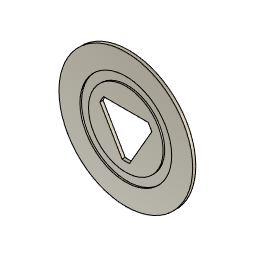
零件1 v3 (Autodesk Fusion 360 design; units mm, degrees)
Autodesk Fusion 360 part; units mm, degrees
sketch "草图1" plane through (0, 0, 0) normal (0, 1, 0) x (1, 0, 0)
  circle A0 centre (0, 0) radius 24.125
  circle A1 centre (0, 0) radius 29.375
  dimension "d1" = 48.25
  dimension "d2" = 58.75
  constraint coincident A0.centre A1.centre
  measures "d1" diameter of A0
  measures "d2" diameter of A1
extrude "拉伸1" add sketch "草图1" along normal blind 0.8 makes body 1
sketch "草图2" plane through (0, 0, 0) normal (0, -1, 0) x (1, 0, 0)
  circle A0 centre (0, 0) radius 24.125
  circle A1 centre (0, 0) radius 29.375
  circle A2 centre (0, 0) radius 43
  line L0 (2.4024, -17.839) -> (16.6502, 6.839)
  line L1 (-16.6502, 6.839) -> (-2.4024, -17.839)
  arc A3 (-14.2478, 11) -> (-16.6502, 6.839) centre (0, 0) ccw
  line L2 (14.2478, 11) -> (-14.2478, 11)
  arc A4 (16.6502, 6.839) -> (14.2478, 11) centre (0, 0) ccw
  arc A5 (-2.4024, -17.839) -> (2.4024, -17.839) centre (0, 0) ccw
  dimension "d5" = 86
  constraint coincident A0.centre A1.centre
  measures "d5" diameter of A2
extrude "拉伸2" add sketch "草图2" along normal blind 2 separate body contours A2 makes body 2
extrude "拉伸3" add sketch "草图2" along normal blind 1 contours A0 | A1 bodies 1 2
extrude "拉伸4" add 1 faces at (-15.1728, -1, -7.9151) along direction (0, -1, 0) up to surface (1 mm away) on bodies 1 bodies 1
sketch "草图3" plane through (0, -2, 0) normal (0, -1, 0) x (1, 0, 0)
  line L0 (16.6502, 6.839) -> (2.4024, -17.839)
  arc A0 (-2.4024, -17.839) -> (2.4024, -17.839) centre (0, 0) ccw
  line L1 (-2.4024, -17.839) -> (-16.6502, 6.839)
  arc A1 (-14.2478, 11) -> (-16.6502, 6.839) centre (0, 0) ccw
  line L2 (-14.2478, 11) -> (14.2478, 11)
  arc A2 (16.6502, 6.839) -> (14.2478, 11) centre (0, 0) ccw
  circle A3 centre (0, 0) radius 43
  circle A4 centre (0, 0) radius 29.5
  circle A5 centre (0, 0) radius 24
  dimension "d12" = 59
  dimension "d13" = 48
  constraint coincident A0.centre A1.centre
  constraint concentric A4 A5
  measures "d12" diameter of A4
  measures "d13" diameter of A5
extrude "拉伸5" cut sketch "草图3" against normal blind 1 contours A4 bodies 1
